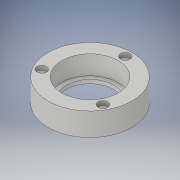
# Autodesk Inventor part: Sensor Deckel293
Saved by Autodesk Inventor 2017 (Build 210142000, 142)
## iProperties
Part Number: Sensor Deckel293
Material: Generisch
Document SubType Name: Modeling
Designer: Harald.Noeske
Density: 1 g/cm^3
Appearance: Vorgabe
Author: Harald.Noeske
Autodesk Inventor part; units mm, degrees
ref_plane "YZ Plane" through (0, 0, 0) normal (1, 0, 0) x (0, 1, 0)
ref_plane "XZ Plane" through (0, 0, 0) normal (0, 1, 0) x (-1, 0, 0)
ref_plane "XY Plane" through (0, 0, 0) normal (0, 0, 1) x (1, 0, 0)
sketch "Skizze1" plane through (0, 0, 0) normal (0, 0, 1) x (1, 0, 0)
  circle A0 centre (0, 0) radius 22
  dimension "d0" = 44
  constraints: 1 centre point, 1 coincident
  measures "d0" diameter of A0
extrude "Extrusion1" add sketch "Skizze1" along normal blind 12
sketch "Skizze2" plane through (0, 0, 12) normal (0, 0, 1) x (1, 0, 0)
  circle A0 centre (0, 18.5) radius 2.525
  point P0 (0, 0)
  dimension "d3" = 5.05
  dimension "d4" = 18.5
  constraints: 1 centre point
  measures "d3" diameter of A0
  measures "d4" distance of A0.centre point (0, 0)
extrude "Extrusion2" cut sketch "Skizze2" against normal blind 2.1
pattern_circular "Runde Anordnung1" count 3 over 360 about axis through (0, 0, 0) along (0, 0, 1) of "Extrusion2"
hole "Bohrung1" at (0, 0, 12) direction (0, 0, -1) diameter 25 depth 12 counterbore diameter 29.5 counterbore depth 10
